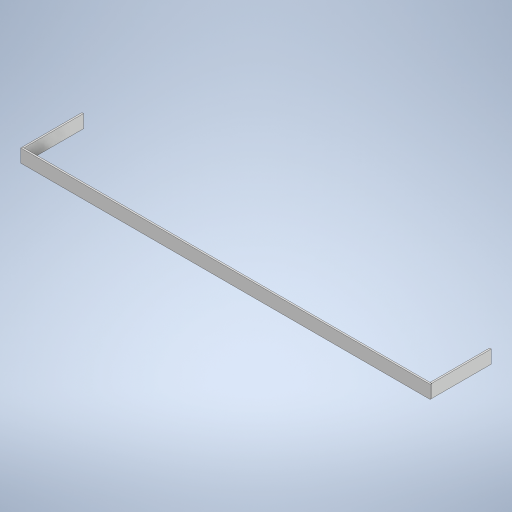
# Autodesk Inventor part: Toe Kick
Saved by Autodesk Inventor 2024 (Build 280153000, 153)
## iProperties
Created: 2023-06-24
Part Number: Toe Kick
Material: Generic
Document SubType Name: Modeling
Designer: 69
Density: 1 g/cm^3
Appearance: Default
Author: 69
Autodesk Inventor part; units mm, degrees
ref_plane "YZ Plane" through (0, 0, 0) normal (1, 0, 0) x (0, 1, 0)
ref_plane "XZ Plane" through (0, 0, 0) normal (0, 1, 0) x (-1, 0, 0)
sketch "Sketch1" plane through (0, 0, 0) normal (0, 0, 1) x (1, 0, 0)
  line L0 (-1498, 0) -> (1498, 0) construction
  line L1 (-1498, 0) -> (-898, 0)
  line L2 (-898, 0) -> (-898, 2068)
  line L3 (-898, 2068) -> (-1498, 2068)
  line L4 (-1498, 2068) -> (-1498, 0)
  line L5 (-898, 0) -> (-498, 0)
  line L6 (-498, 0) -> (-498, 816)
  line L7 (-498, 816) -> (-898, 816)
  line L8 (-898, 816) -> (-898, 0)
  line L9 (-498, 0) -> (102, 0)
  line L10 (102, 0) -> (102, 816)
  line L11 (102, 816) -> (-498, 816)
  line L12 (-498, 816) -> (-498, 0)
  line L13 (102, 0) -> (698, 0)
  line L14 (698, 0) -> (698, 668)
  line L15 (698, 668) -> (102, 668)
  line L16 (102, 668) -> (102, 0)
  line L17 (698, 0) -> (1498, 0)
  line L18 (1498, 0) -> (1498, 816)
  line L19 (1498, 816) -> (698, 816)
  line L20 (698, 816) -> (698, 0)
  line L21 (-1498, 0) -> (1498, 0)
  line L22 (1498, 0) -> (1498, 96)
  line L23 (1498, 96) -> (-1498, 96)
  line L24 (-1498, 96) -> (-1498, 0)
  line L25 (-898, 816) -> (1498, 816)
  line L26 (1498, 816) -> (1498, 832)
  line L27 (1498, 832) -> (-898, 832)
  line L28 (-898, 832) -> (-898, 816)
  line L29 (-898, 1972) -> (-498, 1972)
  line L30 (-498, 1972) -> (-498, 1372)
  line L31 (-498, 1372) -> (-898, 1372)
  line L32 (-898, 1372) -> (-898, 1972)
  line L33 (698, 1972) -> (1498, 1972)
  line L34 (1498, 1972) -> (1498, 1372)
  line L35 (1498, 1372) -> (698, 1372)
  line L36 (698, 1372) -> (698, 1972)
  line L37 (698, 1372) -> (98, 1372)
  line L38 (98, 1372) -> (98, 1972)
  line L39 (98, 1972) -> (698, 1972)
  line L40 (698, 1972) -> (698, 1372)
  line L41 (-498, 1372) -> (98, 1372)
  line L42 (-498, 1372) -> (-275, 1637.7611)
  line L43 (98, 1372) -> (-125, 1637.7611)
  line L44 (-275, 1637.7611) -> (-125, 1637.7611)
  line L45 (-125, 1637.7611) -> (-125, 2068)
  line L46 (-125, 2068) -> (-275, 2068)
  line L47 (-275, 2068) -> (-275, 1637.7611)
  line L48 (1098, 816) -> (1098, 96)
  line L49 (-198, 816) -> (-198, 96)
  line L50 (-898, 668) -> (-498, 668)
  line L51 (-1498, 520) -> (-898, 520)
  line L52 (-1498, 1579) -> (-898, 1579)
  line L53 (398, 1972) -> (398, 1372)
  line L54 (1098, 1972) -> (1098, 1372)
  line L55 (698, 1876) -> (1498, 1876)
  line L56 (698, 1468) -> (1498, 1468)
  line L57 (-1498, 1049.5) -> (-898, 1049.5)
  point P0 (0, 0)
  point P1 (0, 0)
  point P2 (0, 0)
  point P3 (-198, 816)
  point P4 (0, 0)
  dimension "d0" = 2996
  dimension "d1" = 600
  dimension "d2" = 2068
  dimension "d3" = 400
  dimension "d4" = 816
  dimension "d5" = 600
  dimension "d6" = 816
  dimension "d7" = 596
  dimension "d8" = 668
  dimension "d9" = 800
  dimension "d10" = 816
  dimension "d11" = 96
  dimension "d12" = 16
  dimension "d13" = 400
  dimension "d14" = 600
  dimension "d15" = 96
  dimension "d16" = 800
  dimension "d17" = 600
  dimension "d18" = 600
  dimension "d19" = 600
  dimension "d20" = 50
  dimension "d21" = 150
  dimension "d22" = 148
  dimension "d23" = 1059
  dimension "d24" = 96
  dimension "d25" = 96
  dimension "d26" = 529.5
  constraints: 116 end point, 22 parallel, 18 point on line, 17 perpendicular, 14 horizontal, 8 midpoint, 4 coincident, 4 horizontal alignment, 2 vertical alignment, 1 equal length
  measures "d0" distance of L0.start L0.end
  measures "d1" distance of L3.end L2.end
  measures "d2" distance of L2.end L1.end
  measures "d3" distance of L7.end L6.end
  measures "d4" distance of L6.end L5.end
  measures "d5" distance of L11.end L10.end
  measures "d6" distance of L9.end L10.end
  measures "d7" distance of L15.end L14.end
  measures "d8" distance of L14.end L13.end
  measures "d9" distance of L19.end L18.end
  measures "d10" distance of L18.end L17.end
  measures "d11" distance of L22.end L21.end
  measures "d12" distance of L26.end L25.end
  measures "d13" distance of L30.end L31.end
  measures "d14" distance of L29.end L30.end
  measures "d15" distance between parallel lines of L3 L29
  measures "d16" distance of L34.end L35.end
  measures "d17" distance of L33.end L34.end
  measures "d18" distance of L38.end L39.end
  measures "d19" distance of L37.end L38.end
  measures "d20" angle of L41 L42
  measures "d21" distance of L43.end L42.end
  measures "d22" distance of L50.start L51.end
  measures "d23" distance between parallel lines of L51 L52
  measures "d24" distance of L33.start L55.start
  measures "d25" distance of L56.start L35.end
  measures "d26" distance between parallel lines of L51 L57
ref_plane "Work Plane1" through (0, 0, 436) normal (0, 0, 1) x (1, 0, 0)
sketch "Sketch2" plane through (0, 0, 436) normal (0, 0, 1) x (1, 0, 0)
  line L0 (1498, 96) -> (-1498, 96) projected
  line L1 (-1498, 96) -> (1498, 96)
  line L2 (1498, 96) -> (1498, 0)
  line L3 (1498, 0) -> (-1498, 0)
  line L4 (-1498, 0) -> (-1498, 96)
  point P0 (0, 0)
  point P1 (-1498, 0)
  constraints: 8 end point, 2 parallel, 1 horizontal, 1 perpendicular
extrude "Extrusion1" add sketch "Sketch2" along normal blind 12
sketch "Sketch3" plane through (0, 0, 0) normal (0, 1, 0) x (-1, 0, 0)
  line L0 (1498, 436) -> (-1498, 436) projected
  line L1 (1498, 436) -> (1486, 436)
  line L2 (1486, 436) -> (1486, 0)
  line L3 (1486, 0) -> (1498, 0)
  line L4 (1498, 0) -> (1498, 436)
  line L5 (-1498, 436) -> (-1486, 436)
  line L6 (-1486, 436) -> (-1486, 0)
  line L7 (-1486, 0) -> (-1498, 0)
  line L8 (-1498, 0) -> (-1498, 436)
  point P0 (0, 0)
  dimension "d30" = 12
  dimension "d31" = 12
  constraints: 16 end point, 4 parallel, 2 horizontal, 2 perpendicular
  measures "d30" distance between parallel lines of L4 L2
  measures "d31" distance between parallel lines of L8 L6
extrude "Extrusion2" add sketch "Sketch3" along normal up to surface (96 mm away) separate body
